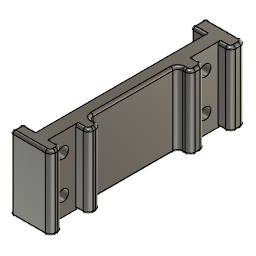
Bracket v2 (Autodesk Fusion 360 design; units mm, degrees)
Autodesk Fusion 360 part; units mm, degrees
sketch "base" plane through (0, 0, 0) normal (0, 0, 1) x (1, 0, 0)
  line L0 (-7.5707, -39.3146) -> (5.4293, -39.3146)
  line L1 (7.4293, -37.3146) -> (7.4293, -36.3146)
  line L2 (-8.5707, -35.3146) -> (-8.5707, -38.3146)
  line L3 (5.4293, -39.3146) -> (2.4293, -39.3146)
  line L4 (2.4293, -34.3146) -> (5.4293, -34.3146)
  line L5 (7.4293, -36.3146) -> (7.4293, -37.3146)
  line L6 (2.4293, -39.3146) -> (-2.5707, -39.3146)
  line L7 (-2.5707, -34.3146) -> (-2.5707, 33.4854)
  line L8 (-2.5707, 39.4854) -> (2.4293, 39.4854)
  line L9 (-7.5707, 39.4854) -> (5.4293, 39.4854)
  line L10 (7.4293, 37.4854) -> (7.4293, 35.4854)
  line L11 (-8.5707, 34.4854) -> (-8.5707, 38.4854)
  line L12 (2.4293, 33.4854) -> (2.4293, 23.1854) construction
  line L13 (2.4293, 23.1854) -> (5.4293, 23.1854)
  line L14 (7.4293, 21.1854) -> (7.4293, 19.1854)
  line L15 (5.4293, 17.1854) -> (4.4293, 17.1854)
  line L16 (2.4293, -34.3146) -> (2.4293, -24.0146) construction
  line L17 (2.4293, -24.0146) -> (5.4293, -24.0146)
  line L18 (7.4293, -22.0146) -> (7.4293, -21.0146)
  line L19 (5.4293, -19.0146) -> (4.4293, -19.0146)
  line L20 (2.4293, -24.0146) -> (2.4293, -34.3146)
  line L21 (5.4293, -34.3146) -> (2.4293, -34.3146)
  line L22 (-2.5707, -34.3146) -> (-7.5707, -34.3146)
  line L23 (2.4293, 33.4854) -> (2.4293, 23.1854)
  line L24 (2.4293, 15.1854) -> (2.4293, -17.0146)
  line L25 (5.4293, 33.4854) -> (2.4293, 33.4854)
  line L26 (-2.5707, 33.4854) -> (-7.5707, 33.4854)
  arc A0 (-7.5707, 39.4854) -> (-8.5707, 38.4854) centre (-7.5707, 38.4854) ccw
  arc A1 (-8.5707, 34.4854) -> (-7.5707, 33.4854) centre (-7.5707, 34.4854) ccw
  arc A2 (-7.5707, -34.3146) -> (-8.5707, -35.3146) centre (-7.5707, -35.3146) ccw
  arc A3 (-8.5707, -38.3146) -> (-7.5707, -39.3146) centre (-7.5707, -38.3146) ccw
  arc A4 (7.4293, 37.4854) -> (5.4293, 39.4854) centre (5.4293, 37.4854) ccw
  arc A5 (5.4293, 33.4854) -> (7.4293, 35.4854) centre (5.4293, 35.4854) ccw
  arc A6 (7.4293, 21.1854) -> (5.4293, 23.1854) centre (5.4293, 21.1854) ccw
  arc A7 (5.4293, 17.1854) -> (7.4293, 19.1854) centre (5.4293, 19.1854) ccw
  arc A8 (4.4293, 17.1854) -> (2.4293, 15.1854) centre (4.4293, 15.1854) ccw
  arc A9 (2.4293, -17.0146) -> (4.4293, -19.0146) centre (4.4293, -17.0146) ccw
  arc A10 (7.4293, -21.0146) -> (5.4293, -19.0146) centre (5.4293, -21.0146) ccw
  arc A11 (5.4293, -24.0146) -> (7.4293, -22.0146) centre (5.4293, -22.0146) ccw
  arc A12 (7.4293, -36.3146) -> (5.4293, -34.3146) centre (5.4293, -36.3146) ccw
  arc A13 (5.4293, -39.3146) -> (7.4293, -37.3146) centre (5.4293, -37.3146) ccw
  point P0 (-8.5707, -39.3146)
  point P1 (-8.5707, -34.3146)
  point P2 (-8.5707, 39.4854)
  point P3 (7.4293, 39.4854)
  point P4 (-8.5707, 33.4854)
  point P5 (7.4293, 23.1854)
  point P6 (2.4293, 17.1854)
  point P7 (7.4293, -24.0146)
  point P8 (2.4293, -19.0146)
  dimension "d2" = 5
  dimension "d4" = 5
  dimension "d5" = 78.8
  dimension "d6" = 16
  dimension "d7" = 6
  dimension "d8" = 6
  dimension "d9" = 10.3
  dimension "d10" = 5
  dimension "d11" = 6
  dimension "d12" = 10.3
  dimension "d13" = 5
  dimension "d14" = 5
  dimension "d15" = 1
  dimension "d16" = 2
  dimension "d17" = 2
  constraint horizontal L0
  constraint vertical L1
  constraint horizontal L21
  constraint vertical L2
  constraint horizontal L3
  constraint horizontal L4
  constraint vertical L5
  constraint horizontal L6
  constraint vertical L7
  constraint horizontal L8
  constraint vertical L23
  constraint horizontal L9
  constraint vertical L10
  constraint horizontal L25
  constraint vertical L11
  constraint collinear L8 L9
  constraint perpendicular L12 L25
  constraint horizontal L13
  constraint vertical L14
  constraint horizontal L15
  constraint perpendicular L4 L16
  constraint horizontal L17
  constraint vertical L18
  constraint horizontal L19
  constraint collinear L20 L23
  constraint coincident L7.start L21
  constraint collinear L21 L22
  constraint collinear L23 L24
  constraint coincident L7.end L25
  constraint collinear L25 L26
  constraint coincident P2 L9
  constraint coincident P2 L11
  constraint tangent L9 A0
  constraint tangent L11 A0
  constraint coincident P4 L11
  constraint coincident P4 L26
  constraint tangent L11 A1
  constraint tangent L26 A1
  constraint equal A0 A1
  constraint coincident P1 L2
  constraint coincident P1 L22
  constraint tangent L2 A2
  constraint tangent L22 A2
  constraint equal A0 A2
  constraint coincident P0 L0
  constraint coincident P0 L2
  constraint tangent L0 A3
  constraint tangent L2 A3
  constraint equal A0 A3
  constraint coincident P3 L9
  constraint coincident P3 L10
  constraint tangent L9 A4
  constraint tangent L10 A4
  constraint tangent L10 A5
  constraint tangent L25 A5
  constraint equal A4 A5
  constraint coincident P5 L13
  constraint coincident P5 L14
  constraint tangent L13 A6
  constraint tangent L14 A6
  constraint equal A4 A6
  constraint tangent L14 A7
  constraint tangent L15 A7
  constraint equal A4 A7
  constraint coincident P6 L15
  constraint coincident P6 L24
  constraint tangent L15 A8
  constraint tangent L24 A8
  constraint equal A4 A8
  constraint coincident P8 L19
  constraint coincident P8 L24
  constraint tangent L19 A9
  constraint tangent L24 A9
  constraint equal A4 A9
  constraint tangent L18 A10
  constraint tangent L19 A10
  constraint equal A4 A10
  constraint coincident P7 L17
  constraint coincident P7 L18
  constraint tangent L17 A11
  constraint tangent L18 A11
  constraint equal A4 A11
  constraint tangent L1 A12
  constraint tangent L21 A12
  constraint equal A4 A12
  constraint tangent L1 A13
  constraint tangent L3 A13
  measures "d2" distance of P0 P1
  measures "d4" distance of L3.end L6.end
  measures "d5" distance of L3.end L8.end
  measures "d6" distance of P2 P3
  measures "d7" distance of P2 P4
  measures "d8" distance of L7 L11
  measures "d9" distance of L12.start L12.end
  measures "d10" distance of L12.end P5
  measures "d11" distance of L12.end P6
  measures "d12" distance of L4.start L16.end
  measures "d13" distance of L16.end P7
  measures "d14" distance of L16.end P8
  measures "d15" radius of A0
  measures "d16" radius of A4
  measures "d17" radius of A13
extrude "Extrude1" add sketch "base" along normal blind 30
sketch "right-holes" plane through (2.4293, 0, 0) normal (1, 0, 0) x (0, 1, 0)
  line L0 (23.1854, 0) -> (33.4854, 0)
  line L1 (33.4854, 0) -> (33.4854, 30)
  line L2 (33.4854, 30) -> (23.1854, 30)
  line L3 (23.1854, 30) -> (23.1854, 0)
  line L4 (33.4854, 30) -> (28.3354, 30)
  line L5 (33.4854, 22.5) -> (33.4854, 30)
  circle A0 centre (28.3354, 22.5) radius 2.25
  line L6 (28.3354, 30) -> (28.3354, 15) construction
  line L7 (23.1854, 15) -> (33.4854, 15) construction
  circle A1 centre (28.3354, 7.5) radius 2.25
  dimension "d20" = 5.15
  dimension "d21" = 7.5
  dimension "d22" = 4.5
  dimension "d23" = 15
  dimension "d24" = 7.5
  constraint horizontal L4
  constraint vertical L5
  constraint coincident L1.end L2.start
  constraint perpendicular L2 L6
  constraint midpoint L3 L7.start
  constraint midpoint L1 L7.end
  constraint symmetric A0 L7 A1
  measures "d20" distance of L1.end L4.end
  measures "d21" distance of L1.end L5.start
  measures "d22" diameter of A0
  measures "d23" distance of L4.end L6.end
  measures "d24" distance of L0 A1.centre
sketch "left-holes" plane through (2.4293, 0, 0) normal (1, 0, 0) x (0, 1, 0)
  line L0 (-34.3146, 0) -> (-24.0146, 0)
  line L1 (-24.0146, 0) -> (-24.0146, 30)
  line L2 (-24.0146, 30) -> (-34.3146, 30)
  line L3 (-34.3146, 30) -> (-34.3146, 0)
  line L4 (-34.3146, 30) -> (-29.1646, 30)
  line L5 (-29.1646, 30) -> (-29.1646, 22.5) construction
  line L6 (-29.1646, 22.5) -> (-34.3146, 22.5) construction
  line L7 (-34.3146, 22.5) -> (-34.3146, 30)
  circle A0 centre (-29.1646, 22.5) radius 2.25
  line L8 (-24.0146, 15) -> (-34.3146, 15) construction
  circle A1 centre (-29.1646, 7.5) radius 2.25
  dimension "d25" = 5.15
  dimension "d26" = 4.5
  constraint horizontal L4
  constraint vertical L5
  constraint horizontal L6
  constraint vertical L7
  constraint coincident L2.end L3.start
  constraint coincident L5.end L6.start
  constraint midpoint L1 L8.start
  constraint midpoint L3 L8.end
  constraint symmetric A0 L8 A1
  measures "d25" distance of L2.end L4.end
  measures "d26" diameter of A0
extrude "Extrude2" cut sketch "left-holes" sketch "right-holes" against normal blind 16 contours A0 | A1 of sketch 2 contours A0 | A1
fillet "Fillet1" radius 1 62 edges at (-5.0707, -34.3146, 30) (-8.2778, -34.6075, 30) (-8.5707, -36.8146, 30) (-8.2778, -39.0217, 30) (-1.0707, -39.3146, 30) (6.8435, -38.7288, 30) (7.4293, -36.8146, 30) (6.8435, -34.9004, 30) (3.9293, -34.3146, 30) (-5.0707, -34.3146, 0) (-8.2778, -34.6075, 0) (-8.5707, -36.8146, 0) (-8.2778, -39.0217, 0) (-1.0707, -39.3146, 0) (6.8435, -38.7288, 0) (7.4293, -36.8146, 0) (6.8435, -34.9004, 0) (3.9293, -34.3146, 0) (3.9293, -24.0146, 0) (6.8435, -23.4288, 0) (7.4293, -21.5146, 0) (6.8435, -19.6004, 0) (4.9293, -19.0146, 0) (3.0151, -18.4288, 0) (2.4293, -0.9146, 0) (3.0151, 16.5996, 0) (4.9293, 17.1854, 0) (6.8435, 17.7712, 0) (7.4293, 20.1854, 0) (6.8435, 22.5996, 0) (3.9293, 23.1854, 0) (3.9293, -24.0146, 30) (6.8435, -23.4288, 30) (7.4293, -21.5146, 30) (6.8435, -19.6004, 30) (4.9293, -19.0146, 30) (3.0151, -18.4288, 30) (2.4293, -0.9146, 30) (3.0151, 16.5996, 30) (4.9293, 17.1854, 30) (6.8435, 17.7712, 30) (7.4293, 20.1854, 30) (6.8435, 22.5996, 30) (3.9293, 23.1854, 30) (3.9293, 33.4854, 30) (6.8435, 34.0712, 30) (7.4293, 36.4854, 30) (6.8435, 38.8996, 30) (-1.0707, 39.4854, 30) (-8.2778, 39.1925, 30) (-8.5707, 36.4854, 30) (-8.2778, 33.7783, 30) (-5.0707, 33.4854, 30) (-5.0707, 33.4854, 0) (-8.2778, 33.7783, 0) (-8.5707, 36.4854, 0) (-8.2778, 39.1925, 0) (-1.0707, 39.4854, 0) (6.8435, 38.8996, 0) (7.4293, 36.4854, 0) (6.8435, 34.0712, 0) (3.9293, 33.4854, 0)
named bodies: "Bracket"
